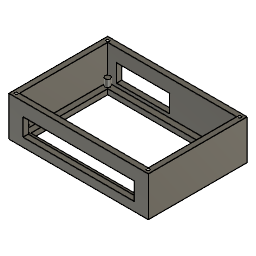
relayboxbottom (Autodesk Fusion 360 design; units mm, degrees)
part number: 2025-12-15-16-26-34-324
Autodesk Fusion 360 part; units mm, degrees
sketch "Sketch1" plane through (0, 0, 0) normal (0, 0, 1) x (1, 0, 0)
  line L0 (39.5, 28) -> (-39.5, 28)
  line L1 (-39.5, 28) -> (-39.5, -28)
  line L2 (-39.5, -28) -> (39.5, -28)
  line L3 (39.5, -28) -> (39.5, 28)
  line L4 (39.5, 28) -> (-39.5, -28) construction
  line L5 (-39.5, 28) -> (39.5, -28) construction
  dimension "d1" = 79
  dimension "d2" = 56
  constraint horizontal L0
  constraint perpendicular L0 L1
  constraint parallel L0 L2
  constraint parallel L1 L3
  constraint coincident L4 origin
  constraint coincident L5 origin
  measures "d1" distance of L1.end L2.end
  measures "d2" distance of L0.end L1.end
extrude "Extrude1" add sketch "Sketch1" along normal blind 22.5
sketch "Sketch2" plane through (0, 0, 22.5) normal (0, 0, 1) x (-1, 0, 0)
  line L0 (-39.5, 28) -> (-39.5, -28)
  line L1 (-39.5, -28) -> (39.5, -28)
  line L2 (39.5, -28) -> (39.5, 28)
  line L3 (39.5, 28) -> (-39.5, 28)
  line L4 (-36.5, -25) -> (36.5, -25)
  line L5 (36.5, -25) -> (36.5, 25)
  line L6 (36.5, 25) -> (-36.5, 25)
  line L7 (-36.5, 25) -> (-36.5, -25)
  line L8 (-36.5, -25) -> (36.5, 25) construction
  line L9 (36.5, -25) -> (-36.5, 25) construction
  dimension "d5" = 73
  dimension "d6" = 50
  constraint horizontal L4
  constraint perpendicular L4 L5
  constraint parallel L4 L6
  constraint parallel L5 L7
  constraint coincident L8 origin
  constraint coincident L9 origin
  measures "d5" distance of L5.end L6.end
  measures "d6" distance of L4.end L5.end
extrude "Extrude2" cut sketch "Sketch2" against normal blind 19.5 contours L4 L5 L6 L7
sketch "Sketch3" plane through (0, 0, 0) normal (0, 0, -1) x (1, 0, 0)
  line L0 (39.5, -28) -> (39.5, 28)
  line L1 (39.5, 28) -> (-39.5, 28)
  line L2 (-39.5, 28) -> (-39.5, -28)
  line L3 (-39.5, -28) -> (39.5, -28)
  line L4 (33.25, 21.75) -> (-33.25, 21.75)
  line L5 (-33.25, 21.75) -> (-33.25, -21.75)
  line L6 (-33.25, -21.75) -> (33.25, -21.75)
  line L7 (33.25, -21.75) -> (33.25, 21.75)
  line L8 (33.25, 21.75) -> (-33.25, -21.75) construction
  line L9 (-33.25, 21.75) -> (33.25, -21.75) construction
  dimension "d9" = 66.5
  dimension "d10" = 43.5
  constraint horizontal L4
  constraint perpendicular L4 L5
  constraint parallel L4 L6
  constraint parallel L5 L7
  constraint coincident L8 origin
  constraint coincident L9 origin
  measures "d9" distance of L5.end L6.end
  measures "d10" distance of L4.end L5.end
sketch "Sketch4" plane through (0, 0, 0) normal (0, 0, -1) x (1, 0, 0)
extrude "Extrude3" cut sketch "Sketch3" against normal blind 3 contours L4 L5 L6 L7
sketch "Sketch5" plane through (0, 0, 3) normal (0, 0, 1) x (-1, 0, 0)
  line L0 (-33.25, 21.75) -> (33.25, 21.75)
  line L1 (33.25, 21.75) -> (33.25, -21.75)
  line L2 (33.25, -21.75) -> (-33.25, -21.75)
  line L3 (-33.25, -21.75) -> (-33.25, 21.75)
  line L4 (-36.5, 25) -> (-36.5, -25)
  line L5 (-36.5, -25) -> (36.5, -25)
  line L6 (36.5, -25) -> (36.5, 25)
  line L7 (36.5, 25) -> (-36.5, 25)
  circle A0 centre (34.875, -23.375) radius 1.5
  dimension "d13" = 3
  dimension "d14" = 1.625
  dimension "d15" = 1.625
  measures "d13" diameter of A0
  measures "d14" distance of L5 A0.centre
  measures "d15" distance of L6 A0.centre
sketch "Sketch6" plane through (0, 0, 3) normal (0, 0, 1) x (-1, 0, 0)
  circle A0 centre (-34.875, -23.375) radius 1.5
  line L0 (-36.5, -25) -> (36.5, -25)
  line L1 (-36.5, 25) -> (-36.5, -25)
  circle A1 centre (-34.875, 23.375) radius 1.5
  line L2 (36.5, 25) -> (-36.5, 25)
  circle A2 centre (34.875, 23.375) radius 1.5
  line L3 (36.5, -25) -> (36.5, 25)
  dimension "d16" = 3
  dimension "d17" = 1.625
  dimension "d18" = 1.625
  dimension "d19" = 3
  dimension "d20" = 1.625
  dimension "d21" = 1.625
  dimension "d25" = 3
  dimension "d26" = 1.625
  dimension "d27" = 1.625
  measures "d16" diameter of A0
  measures "d17" distance of A0.centre L0
  measures "d18" distance of A0.centre L1
  measures "d19" diameter of A1
  measures "d20" distance of L1 A1.centre
  measures "d21" distance of A1.centre L2
  measures "d25" diameter of A2
  measures "d26" distance of L2 A2.centre
  measures "d27" distance of A2.centre L3
sketch "Sketch7" plane through (0, 0, 3) normal (0, 0, 1) x (-1, 0, 0)
  circle A0 centre (34.875, 23.375) radius 1.55
  line L0 (36.5, 25) -> (-36.5, 25)
  line L1 (36.5, -25) -> (36.5, 25)
  dimension "d22" = 3.1
  dimension "d23" = 1.625
  dimension "d24" = 1.625
  measures "d22" diameter of A0
  measures "d23" distance of A0.centre L0
  measures "d24" distance of A0.centre L1
extrude "Extrude4" add sketch "Sketch5" sketch "Sketch7" sketch "Sketch6" along normal blind 4 contours A0 of sketch 2 of sketch 3 contours A0 | A1
sketch "Sketch8" plane through (0, -28, 0) normal (0, -1, 0) x (1, 0, 0)
  line L0 (-39.5, 0) -> (39.5, 0)
  line L1 (39.5, 0) -> (39.5, 22.5)
  line L2 (39.5, 22.5) -> (-39.5, 22.5)
  line L3 (-39.5, 22.5) -> (-39.5, 0)
  line L4 (31.5, 15) -> (-31.5, 15)
  line L5 (-31.5, 15) -> (-31.5, 5)
  line L6 (-31.5, 5) -> (31.5, 5)
  line L7 (31.5, 5) -> (31.5, 15)
  line L8 (31.5, 15) -> (-31.5, 5) construction
  line L9 (-31.5, 15) -> (31.5, 5) construction
  point P0 (0, 10)
  dimension "d30" = 63
  dimension "d31" = 10
  dimension "d33" = 15
  constraint horizontal L4
  constraint perpendicular L4 L5
  constraint parallel L4 L6
  constraint parallel L5 L7
  constraint coincident L8 P0
  constraint coincident L9 P0
  measures "d30" distance of L5.end L6.end
  measures "d31" distance of L4.end L5.end
  measures "d33" distance of L0 L4
extrude "Extrude5" cut sketch "Sketch8" against normal blind 3 contours L4 L5 L6 L7
sketch "Sketch9" plane through (0, 28, 0) normal (0, 1, 0) x (-1, 0, 0)
  line L0 (-39.5, 0) -> (39.5, 0)
  line L1 (39.5, 0) -> (39.5, 22.5)
  line L2 (39.5, 22.5) -> (-39.5, 22.5)
  line L3 (-39.5, 22.5) -> (-39.5, 0)
  line L4 (31.5, 15) -> (1.5, 15)
  line L5 (1.5, 15) -> (1.5, 5)
  line L6 (1.5, 5) -> (31.5, 5)
  line L7 (31.5, 5) -> (31.5, 15)
  line L8 (31.5, 15) -> (1.5, 5) construction
  line L9 (1.5, 15) -> (31.5, 5) construction
  point P0 (16.5, 10)
  dimension "d36" = 30
  dimension "d37" = 10
  dimension "d38" = 8
  dimension "d39" = 15
  constraint horizontal L4
  constraint perpendicular L4 L5
  constraint parallel L4 L6
  constraint parallel L5 L7
  constraint coincident L8 P0
  constraint coincident L9 P0
  measures "d36" distance of L5.end L6.end
  measures "d37" distance of L4.end L5.end
  measures "d38" distance of L1 L7
  measures "d39" distance of L0 L4
extrude "Extrude6" cut sketch "Sketch9" against normal blind 3 contours L4 L5 L6 L7
sketch "Sketch11" plane through (0, 0, 22.5) normal (0, 0, 1) x (-1, 0, 0)
  line L0 (36.5, -25) -> (-36.5, -25)
  line L1 (-36.5, -25) -> (-36.5, 25)
  line L2 (-36.5, 25) -> (36.5, 25)
  line L3 (36.5, 25) -> (36.5, -25)
  line L4 (-39.5, 28) -> (-39.5, -28)
  line L5 (-39.5, -28) -> (39.5, -28)
  line L6 (39.5, -28) -> (39.5, 28)
  line L7 (39.5, 28) -> (-39.5, 28)
  circle A0 centre (37.375, -25.875) radius 1
  circle A1 centre (37.375, 25.875) radius 1
  circle A2 centre (-37.375, 25.875) radius 1
  circle A3 centre (-37.375, -25.875) radius 1
  dimension "d56" = 2
  dimension "d57" = 2
  dimension "d58" = 2
  dimension "d59" = 2
  dimension "d60" = 2.125
  dimension "d61" = 2.125
  dimension "d62" = 2.125
  dimension "d63" = 2.125
  dimension "d64" = 2.125
  dimension "d65" = 2.125
  dimension "d66" = 2.125
  dimension "d67" = 2.125
  measures "d56" diameter of A0
  measures "d57" diameter of A1
  measures "d58" diameter of A2
  measures "d59" diameter of A3
  measures "d60" distance of L5 A0.centre
  measures "d61" distance of L6 A0.centre
  measures "d62" distance of L5 A3.centre
  measures "d63" distance of L4 A3.centre
  measures "d64" distance of L4 A2.centre
  measures "d65" distance of L7 A2.centre
  measures "d66" distance of L7 A1.centre
  measures "d67" distance of L6 A1.centre
hole "Hole1" at (-37.375, 25.875, 22.5) at (37.375, 25.875, 22.5) at (37.375, -25.875, 22.5) at (-37.375, -25.875, 22.5) direction (0, 0, -1) diameter 1.6256 depth 5 tip angle 180
thread "Thread1" "ISO Metric profile 2.0 M2x0.4 M2x0.4 6H" thread offset 0 thread depth 5.9436
